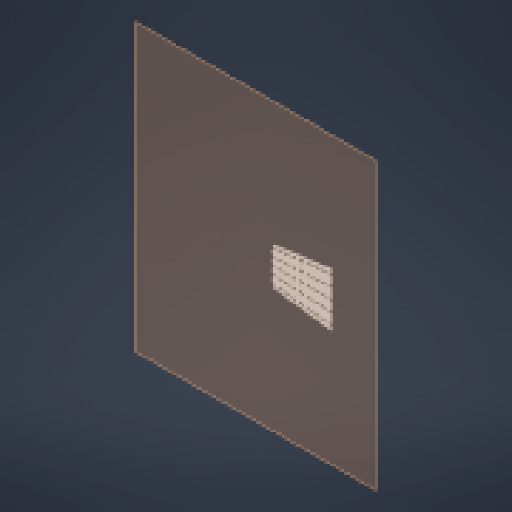
# Autodesk Inventor part: PCB
Saved by Autodesk Inventor 2023 (Build 270158000, 158)
## iProperties
Created: 2022-07-05
Part Number: PCB
Material: Generic
Document SubType Name: Modeling
Designer: FizzyApple12
Density: 1 g/cm^3
Appearance: Default
Author: FizzyApple12
Autodesk Inventor part; units mm, degrees
(part 1 of 2)
ref_plane "YZ Plane" through (0, 0, 0) normal (1, 0, 0) x (0, 1, 0)
ref_plane "XZ Plane" through (0, 0, 0) normal (0, 1, 0) x (-1, 0, 0)
ref_plane "XY Plane" through (0, 0, 0) normal (0, 0, 1) x (1, 0, 0)
ref_plane "Work Plane1" through (0, 0, 0) normal (0, 0, 1) x (1, 0, 0)
sketch "Sketch1" plane through (0, 0, 0) normal (0, 0, 1) x (1, 0, 0)
  line L0 (-101.355, 3.175) -> (-101.355, -3.175) construction
  line L1 (-101.355, -3.175) -> (-123.1468, -3.175) construction
  line L2 (-123.1468, -3.175) -> (-123.1468, 3.175) construction
  line L3 (-123.1468, 3.175) -> (-101.355, 3.175) construction
  line L4 (-101.2199, -3.175) -> (-101.2199, 3.175) construction
  line L5 (-101.2199, 3.175) -> (-5.5562, 3.175) construction
  line L6 (-5.5562, 3.175) -> (-5.5562, -3.175) construction
  line L7 (-5.5562, -3.175) -> (-101.2199, -3.175) construction
  line L8 (120.7237, 3.175) -> (120.7237, -3.175) construction
  line L9 (120.7237, -3.175) -> (5.5563, -3.175) construction
  line L10 (5.5563, -3.175) -> (5.5563, 3.175) construction
  line L11 (5.5563, 3.175) -> (120.7237, 3.175) construction
  line L12 (127.5011, 3.175) -> (127.5011, -3.175) construction
  line L13 (127.5011, -3.175) -> (124.6594, -3.175) construction
  line L14 (124.6594, -3.175) -> (124.6594, 3.175) construction
  line L15 (124.6594, 3.175) -> (127.5011, 3.175) construction
  line L16 (-119.8652, 80.4661) -> (-119.8652, 69.6849) construction
  line L17 (-119.8652, 69.6849) -> (-123.5942, 69.2692) construction
  line L18 (-123.5942, 69.2692) -> (-123.5942, 79.942) construction
  line L19 (-123.5942, 79.942) -> (-119.8652, 80.4661) construction
  line L20 (-119.8652, 63.1931) -> (-119.8652, 36.045) construction
  line L21 (-119.8652, 36.045) -> (-123.5942, 35.8394) construction
  line L22 (-123.5942, 35.8394) -> (-123.5942, 62.7773) construction
  line L23 (-123.5942, 62.7773) -> (-119.8652, 63.1931) construction
  line L24 (-119.8652, 29.66) -> (-119.8652, 3.175) construction
  line L25 (-119.8652, 3.175) -> (-123.5942, 3.175) construction
  line L26 (-123.5942, 3.175) -> (-123.5942, 29.4545) construction
  line L27 (-123.5942, 29.4545) -> (-119.8652, 29.66) construction
  line L28 (-119.8652, -3.175) -> (-119.8652, -29.66) construction
  line L29 (-119.8652, -29.66) -> (-123.5942, -29.4545) construction
  line L30 (-123.5942, -29.4545) -> (-123.5942, -3.175) construction
  line L31 (-123.5942, -3.175) -> (-119.8652, -3.175) construction
  line L32 (-119.8652, -36.045) -> (-119.8652, -63.1931) construction
  line L33 (-119.8652, -63.1931) -> (-123.5942, -62.7773) construction
  line L34 (-123.5942, -62.7773) -> (-123.5942, -35.8394) construction
  line L35 (-123.5942, -35.8394) -> (-119.8652, -36.045) construction
  line L36 (-119.8652, -69.6849) -> (-119.8652, -80.4661) construction
  line L37 (-119.8652, -80.4661) -> (-123.5942, -79.942) construction
  line L38 (-123.5942, -79.942) -> (-123.5942, -69.2692) construction
  line L39 (-123.5942, -69.2692) -> (-119.8652, -69.6849) construction
  line L40 (-109.6354, -30.2239) -> (-110.9009, -36.5392) construction
  line L41 (-110.9009, -36.5392) -> (-123.1468, -35.8641) construction
  line L42 (-123.1468, -35.8641) -> (-123.1468, -29.4791) construction
  line L43 (-123.1468, -29.4791) -> (-109.6354, -30.2239) construction
  line L44 (-104.0884, -30.5297) -> (-105.3539, -36.8449) construction
  line L45 (-105.3539, -36.8449) -> (-109.4238, -36.6206) construction
  line L46 (-109.4238, -36.6206) -> (-109.4238, -30.2356) construction
  line L47 (-109.4238, -30.2356) -> (-104.0884, -30.5297) construction
  line L48 (-101.2199, -37.0728) -> (-101.2199, -30.6879) construction
  line L49 (-101.2199, -30.6879) -> (-6.4561, -35.9117) construction
  line L50 (-6.4561, -35.9117) -> (-6.8056, -42.2774) construction
  line L51 (-6.8056, -42.2774) -> (-101.2199, -37.0728) construction
  line L52 (118.4505, -42.7972) -> (118.5665, -49.1886) construction
  line L53 (118.5665, -49.1886) -> (4.2901, -42.8891) construction
  line L54 (4.2901, -42.8891) -> (4.6396, -36.5234) construction
  line L55 (4.6396, -36.5234) -> (118.4505, -42.7972) construction
  line L56 (-115.3903, -68.5048) -> (-116.0414, -70.1112) construction
  line L57 (-116.0414, -70.1112) -> (-123.1468, -69.3191) construction
  line L58 (-123.1468, -69.3191) -> (-123.1468, -62.8272) construction
  line L59 (-123.1468, -62.8272) -> (-115.3903, -63.6919) construction
  line L60 (-115.3903, -63.6919) -> (-115.3903, -68.5048) construction
  line L61 (-106.228, -71.2052) -> (-103.7108, -64.994) construction
  line L62 (-103.7108, -64.994) -> (-7.378, -75.7333) construction
  line L63 (-7.378, -75.7333) -> (-8.0816, -82.1467) construction
  line L64 (-8.0816, -82.1467) -> (-106.228, -71.2052) construction
  line L65 (121.8551, -96.6323) -> (123.9264, -90.3713) construction
  line L66 (123.9264, -90.3713) -> (132.9258, -91.3746) construction
  line L67 (132.9258, -91.3746) -> (132.9258, -93.8676) construction
  line L68 (132.9258, -93.8676) -> (131.3752, -97.6936) construction
  line L69 (131.3752, -97.6936) -> (121.8551, -96.6323) construction
  line L70 (119.8868, -95.8185) -> (119.9083, -96.4152) construction
  line L71 (119.9083, -96.4152) -> (119.6563, -96.3871) construction
  line L72 (119.6563, -96.3871) -> (119.8868, -95.8185) construction
  line L73 (110.999, -88.9302) -> (110.999, -95.422) construction
  line L74 (110.999, -95.422) -> (-1.3664, -82.8953) construction
  line L75 (-1.3664, -82.8953) -> (-0.6628, -76.4819) construction
  line L76 (-0.6628, -76.4819) -> (110.999, -88.9302) construction
  line L77 (132.9258, -115.9918) -> (132.9258, -119.2788) construction
  line L78 (132.9258, -119.2788) -> (129.106, -118.742) construction
  line L79 (129.106, -118.742) -> (130.6728, -115.6752) construction
  line L80 (130.6728, -115.6752) -> (132.9258, -115.9918) construction
  line L81 (117.7113, -116.5113) -> (117.4113, -117.0985) construction
  line L82 (117.4113, -117.0985) -> (69.7285, -110.3974) construction
  ellipse E0 centre (66.7779, -107.4466) end of major axis (64.6445, -122.6275) minor radius 3.3782 (69.7285, -110.3974) -> (70.2228, -107.1799) ccw construction
  line L83 (70.2228, -107.1799) -> (117.7113, -113.8536) construction
  line L84 (117.7113, -113.8536) -> (117.7113, -116.5113) construction
  line L85 (-122.3603, -80.1155) -> (-123.1468, -81.6549) construction
  line L86 (-123.1468, -81.6549) -> (-123.1468, -80.0049) construction
  line L87 (-123.1468, -80.0049) -> (-122.3603, -80.1155) construction
  line L88 (-107.9322, -85.4301) -> (-107.9322, -82.1431) construction
  line L89 (-107.9322, -82.1431) -> (-61.1887, -88.7121) construction
  ellipse E1 centre (-59.8413, -98.3515) end of major axis (-61.9747, -113.5324) minor radius 3.3782 (-61.1887, -88.7121) -> (-62.0608, -91.8766) ccw construction
  line L90 (-62.0608, -91.8766) -> (-107.9322, -85.4301) construction
  line L91 (63.1283, -109.4699) -> (-55.9232, -92.7391) construction
  ellipse E2 centre (-59.8413, -98.3515) end of major axis (-61.9747, -113.5324) minor radius 3.3782 (-55.9232, -92.7391) -> (-55.8893, -89.4569) ccw construction
  line L92 (-55.8893, -89.4569) -> (63.54, -106.2407) construction
  ellipse E3 centre (66.7779, -107.4466) end of major axis (64.6445, -122.6275) minor radius 3.3782 (63.54, -106.2407) -> (63.1283, -109.4699) ccw construction
  line L93 (-110.9009, 36.5392) -> (-109.6354, 30.2239) construction
  line L94 (-109.6354, 30.2239) -> (-123.1468, 29.4791) construction
  line L95 (-123.1468, 29.4791) -> (-123.1468, 35.8641) construction
  line L96 (-123.1468, 35.8641) -> (-110.9009, 36.5392) construction
  line L97 (-105.3539, 36.8449) -> (-104.0884, 30.5297) construction
  line L98 (-104.0884, 30.5297) -> (-109.4238, 30.2356) construction
  line L99 (-109.4238, 30.2356) -> (-109.4238, 36.6206) construction
  line L100 (-109.4238, 36.6206) -> (-105.3539, 36.8449) construction
  line L101 (-101.2199, 30.6879) -> (-101.2199, 37.0728) construction
  line L102 (-101.2199, 37.0728) -> (-6.8056, 42.2774) construction
  line L103 (-6.8056, 42.2774) -> (-6.4561, 35.9117) construction
  line L104 (-6.4561, 35.9117) -> (-101.2199, 30.6879) construction
  line L105 (118.5665, 49.1886) -> (118.4505, 42.7972) construction
  line L106 (118.4505, 42.7972) -> (4.6396, 36.5234) construction
  line L107 (4.6396, 36.5234) -> (4.2901, 42.8891) construction
  line L108 (4.2901, 42.8891) -> (118.5665, 49.1886) construction
  line L109 (-116.0414, 70.1112) -> (-115.3903, 68.5048) construction
  line L110 (-115.3903, 68.5048) -> (-115.3903, 63.6919) construction
  line L111 (-115.3903, 63.6919) -> (-123.1468, 62.8272) construction
  line L112 (-123.1468, 62.8272) -> (-123.1468, 69.3191) construction
  line L113 (-123.1468, 69.3191) -> (-116.0414, 70.1112) construction
  line L114 (-103.7108, 64.994) -> (-106.228, 71.2052) construction
  line L115 (-106.228, 71.2052) -> (-8.0816, 82.1467) construction
  line L116 (-8.0816, 82.1467) -> (-7.378, 75.7333) construction
  line L117 (-7.378, 75.7333) -> (-103.7108, 64.994) construction
  line L118 (123.9264, 90.3713) -> (121.8551, 96.6323) construction
  line L119 (121.8551, 96.6323) -> (131.3752, 97.6936) construction
  line L120 (131.3752, 97.6936) -> (132.9258, 93.8676) construction
  line L121 (132.9258, 93.8676) -> (132.9258, 91.3746) construction
  line L122 (132.9258, 91.3746) -> (123.9264, 90.3713) construction
  line L123 (119.9083, 96.4152) -> (119.8868, 95.8185) construction
  line L124 (119.8868, 95.8185) -> (119.6563, 96.3871) construction
  line L125 (119.6563, 96.3871) -> (119.9083, 96.4152) construction
  line L126 (110.999, 95.422) -> (110.999, 88.9302) construction
  line L127 (110.999, 88.9302) -> (-0.6628, 76.4819) construction
  line L128 (-0.6628, 76.4819) -> (-1.3664, 82.8953) construction
  line L129 (-1.3664, 82.8953) -> (110.999, 95.422) construction
  line L130 (132.9258, 119.2788) -> (132.9258, 115.9918) construction
  line L131 (132.9258, 115.9918) -> (130.6728, 115.6752) construction
  line L132 (130.6728, 115.6752) -> (129.106, 118.742) construction
  line L133 (129.106, 118.742) -> (132.9258, 119.2788) construction
  line L134 (117.4113, 117.0985) -> (117.7113, 116.5113) construction
  line L135 (117.7113, 116.5113) -> (117.7113, 113.8536) construction
  line L136 (117.7113, 113.8536) -> (70.2228, 107.1799) construction
  ellipse E4 centre (66.7779, 107.4466) end of major axis (64.6445, 122.6275) minor radius 3.3782 (70.2228, 107.1799) -> (69.7285, 110.3974) ccw construction
  line L137 (69.7285, 110.3974) -> (117.4113, 117.0985) construction
  line L138 (-123.1468, 81.6549) -> (-122.3603, 80.1155) construction
  line L139 (-122.3603, 80.1155) -> (-123.1468, 80.0049) construction
  line L140 (-123.1468, 80.0049) -> (-123.1468, 81.6549) construction
  line L141 (-107.9322, 82.1431) -> (-107.9322, 85.4301) construction
  line L142 (-107.9322, 85.4301) -> (-62.0608, 91.8766) construction
  ellipse E5 centre (-59.8413, 98.3515) end of major axis (-61.9747, 113.5324) minor radius 3.3782 (-62.0608, 91.8766) -> (-61.1887, 88.7121) ccw construction
  line L143 (-61.1887, 88.7121) -> (-107.9322, 82.1431) construction
  line L144 (63.54, 106.2407) -> (-55.8893, 89.4569) construction
  ellipse E6 centre (-59.8413, 98.3515) end of major axis (-61.9747, 113.5324) minor radius 3.3782 (-55.8893, 89.4569) -> (-55.9232, 92.7391) ccw construction
  line L145 (-55.9232, 92.7391) -> (63.1283, 109.4699) construction
  ellipse E7 centre (66.7779, 107.4466) end of major axis (64.6445, 122.6275) minor radius 3.3782 (63.1283, 109.4699) -> (63.54, 106.2407) ccw construction
  line L146 (0.1826, -83.068) -> (3.9116, -83.4837) construction
  line L147 (3.9116, -83.4837) -> (3.9116, -97.8609) construction
  line L148 (3.9116, -97.8609) -> (0.1826, -97.3369) construction
  line L149 (0.1826, -97.3369) -> (0.1826, -83.068) construction
  line L150 (3.9116, 83.4837) -> (0.1826, 83.068) construction
  line L151 (0.1826, 83.068) -> (0.1826, 97.3369) construction
  line L152 (0.1826, 97.3369) -> (3.9116, 97.8609) construction
  line L153 (3.9116, 97.8609) -> (3.9116, 83.4837) construction
  line L154 (3.9116, 45.8053) -> (0.1826, 45.5997) construction
  line L155 (0.1826, 45.5997) -> (0.1826, 76.5762) construction
  line L156 (0.1826, 76.5762) -> (3.9116, 76.9919) construction
  line L157 (3.9116, 76.9919) -> (3.9116, 45.8053) construction
  line L158 (3.9116, 6.096) -> (0.1826, 6.096) construction
  line L159 (0.1826, 6.096) -> (0.1826, 33.3406) construction
  line L160 (0.1826, 33.3406) -> (3.9116, 33.5461) construction
  line L161 (3.9116, 33.5461) -> (3.9116, 6.096) construction
  line L162 (3.9116, -33.5461) -> (0.1826, -33.3406) construction
  line L163 (0.1826, -33.3406) -> (0.1826, -6.096) construction
  line L164 (0.1826, -6.096) -> (3.9116, -6.096) construction
  line L165 (3.9116, -6.096) -> (3.9116, -33.5461) construction
  line L166 (0.1826, -45.5997) -> (3.9116, -45.8053) construction
  line L167 (3.9116, -45.8053) -> (3.9116, -76.9919) construction
  line L168 (3.9116, -76.9919) -> (0.1826, -76.5762) construction
  line L169 (0.1826, -76.5762) -> (0.1826, -45.5997) construction
  line L170 (129.6442, 43.4142) -> (133.3733, 43.6198) construction
  line L171 (133.3733, 43.6198) -> (133.3733, 3.175) construction
  line L172 (133.3733, 3.175) -> (133.2928, 3.175) construction
  ellipse E8 centre (131.0926, 0) end of major axis (137.5337, 0) minor radius 3.3782 (133.2928, 3.175) -> (129.6442, 3.2917) ccw construction
  line L173 (129.6442, 3.2917) -> (129.6442, 43.4142) construction
  line L174 (133.3733, -43.6198) -> (129.6442, -43.4142) construction
  line L175 (129.6442, -43.4142) -> (129.6442, -3.2917) construction
  ellipse E9 centre (131.0926, 0) end of major axis (137.5337, 0) minor radius 3.3782 (129.6442, -3.2917) -> (133.2928, -3.175) ccw construction
  line L176 (133.2928, -3.175) -> (133.3733, -3.175) construction
  line L177 (133.3733, -3.175) -> (133.3733, -43.6198) construction
  line L178 (133.3733, -91.4245) -> (129.6442, -91.0088) construction
  line L179 (129.6442, -91.0088) -> (129.6442, -49.7992) construction
  line L180 (129.6442, -49.7992) -> (133.3733, -50.0048) construction
  line L181 (133.3733, -50.0048) -> (133.3733, -91.4245) construction
  line L182 (129.6442, 91.0088) -> (133.3733, 91.4245) construction
  line L183 (133.3733, 91.4245) -> (133.3733, 50.0048) construction
  line L184 (133.3733, 50.0048) -> (129.6442, 49.7992) construction
  line L185 (129.6442, 49.7992) -> (129.6442, 91.0088) construction
  line L186 (133.3733, 116.0547) -> (133.3733, 105.7455) construction
  ellipse E10 centre (131.0926, 102.5862) end of major axis (137.5337, 102.5862) minor radius 3.3782 (133.3733, 105.7455) -> (129.6442, 105.8778) ccw construction
  line L187 (129.6442, 105.8778) -> (129.6442, 115.5306) construction
  line L188 (129.6442, 115.5306) -> (133.3733, 116.0547) construction
  line L189 (133.3733, -92.7634) -> (133.3733, -99.4268) construction
  ellipse E11 centre (131.0926, -102.5862) end of major axis (137.5337, -102.5862) minor radius 3.3782 (133.3733, -99.4268) -> (129.6442, -99.2945) ccw construction
  line L190 (129.6442, -99.2945) -> (129.6442, -97.5006) construction
  line L191 (129.6442, -97.5006) -> (131.3752, -97.6936) construction
  line L192 (131.3752, -97.6936) -> (133.3733, -92.7634) construction
  line L193 (133.3733, -105.7455) -> (133.3733, -116.0547) construction
  line L194 (133.3733, -116.0547) -> (129.6442, -115.5306) construction
  line L195 (129.6442, -115.5306) -> (129.6442, -105.8778) construction
  ellipse E12 centre (131.0926, -102.5862) end of major axis (137.5337, -102.5862) minor radius 3.3782 (129.6442, -105.8778) -> (133.3733, -105.7455) ccw construction
  line L196 (131.3752, 97.6936) -> (129.6442, 97.5006) construction
  line L197 (129.6442, 97.5006) -> (129.6442, 99.2945) construction
  ellipse E13 centre (131.0926, 102.5862) end of major axis (137.5337, 102.5862) minor radius 3.3782 (129.6442, 99.2945) -> (133.3733, 99.4268) ccw construction
  line L198 (133.3733, 99.4268) -> (133.3733, 92.7634) construction
  line L199 (133.3733, 92.7634) -> (131.3752, 97.6936) construction
  line L200 (-119.8652, 29.66) -> (129.6442, 43.4142)
  line L201 (-119.8652, -36.045) -> (129.6442, -49.7992)
  line L202 (-119.8652, -29.66) -> (129.6442, -43.4142)
  line L203 (-119.8652, 3.175) -> (129.6442, 3.175)
  line L204 (-119.8652, -3.175) -> (129.6442, -3.175)
  line L205 (-119.8652, 36.045) -> (129.6442, 49.7992)
  line L206 (-119.8652, -69.6849) -> (129.6442, -97.5006)
  line L207 (-119.8652, -63.1931) -> (129.6442, -91.0088)
  line L208 (-119.8652, 63.1931) -> (129.6442, 91.0088)
  line L209 (-119.8652, 69.6849) -> (129.6442, 97.5006)
  line L210 (129.6442, 43.4142) -> (129.6442, 3.175)
  line L211 (129.6442, 91.0088) -> (129.6442, 49.7992)
  line L212 (129.6442, -3.175) -> (129.6442, -43.4142)
  line L213 (129.6442, -49.7992) -> (129.6442, -91.0088)
  line L214 (-119.8652, -36.045) -> (-119.8652, -63.1931)
  line L215 (-119.8652, 29.66) -> (-119.8652, 3.175)
  line L216 (-119.8652, -3.175) -> (-119.8652, -29.66)
  line L217 (-119.8652, 63.1931) -> (-119.8652, 36.045)
  line L218 (129.6442, -115.5306) -> (-119.8652, -80.4661)
  line L219 (129.6442, 115.5306) -> (-119.8652, 80.4661)
  line L220 (129.6442, 115.5306) -> (129.6442, 97.5006)
  line L221 (-119.8652, -80.4661) -> (-119.8652, -69.6849)
  line L222 (129.6442, -115.5306) -> (129.6442, -97.5006)
  line L223 (0.1826, 97.3369) -> (0.1826, -97.3369)
  line L224 (3.9116, 97.8609) -> (3.9116, -97.8609)
  line L225 (-119.8652, 80.4661) -> (-119.8652, 69.6849)
  point P0 (0, 0)
  point P1 (4.8895, -42.9221)
  point P2 (4.8895, -36.5371)
  point P3 (4.8895, -77.1009)
  point P4 (4.8895, -83.5928)
  point P5 (4.8895, -3.175)
  point P6 (4.8895, 3.175)
  point P7 (4.8895, 42.9221)
  point P8 (4.8895, 77.1009)
  point P9 (4.8895, 83.5928)
  point P10 (129.6442, -70.404)
  point P11 (129.6442, 70.404)
  point P12 (129.6442, 23.2946)
  point P13 (129.6442, -23.2946)
  point P14 (-119.8652, 49.619)
  point P15 (-119.8652, 16.4175)
  point P16 (-119.8652, -16.4175)
  point P17 (-119.8652, -49.619)
  point P18 (4.8895, -97.9984)
  point P19 (4.8895, 97.9984)
  point P20 (129.6442, 106.5156)
  point P21 (129.6442, -106.5156)
  point P22 (-119.8652, -75.0755)
  point P23 (0.1826, 0)
  point P24 (3.9116, 0)
  point P25 (-119.8652, 75.0755)
  point P26 (3.9116, 83.4837)
  point P27 (3.9116, 76.9919)
  point P28 (3.9116, 42.8682)
  point P29 (3.9116, 36.4832)
  point P30 (3.9116, 3.175)
  point P31 (3.9116, -3.175)
  point P32 (3.9116, -36.4832)
  point P33 (3.9116, -42.8682)
  point P34 (3.9116, -76.9919)
  point P35 (3.9116, -83.4837)
  point P36 (0.1826, -83.068)
  point P37 (0.1826, -76.5762)
  point P38 (0.1826, -42.6626)
  point P39 (0.1826, -36.2777)
  point P40 (0.1826, -3.175)
  point P41 (0.1826, 3.175)
  point P42 (0.1826, 36.2777)
  point P43 (0.1826, 42.6626)
  point P44 (0.1826, 76.5762)
  point P45 (0.1826, 83.068)
  constraints: 452 end point, 70 point on line, 70 vertical, 33 midpoint, 26 collinear, 14 horizontal, 398 other
extrude "Extrusion1" add sketch "Sketch1" against normal blind 1.6 contours L200 L223 L203 L215 | L200 L210 L203 L224 | L205 L217 L208 L223 | L224 L208 L211 L205 | L223 L202 L216 L204 | L204 L212 L202 L224 | L209 L225 L219 L223 | L224 L219 L220 L209 | L223 L207 L214 L201 | L201 L213 L207 L224 | L223 L218 L221 L206 | L206 L222 L218 L224
sketch "Sketch2" plane through (0, 0, -1.6) normal (0, 0, -1) x (-1, 0, 0)
  line L0 (-4.8972, -83.8832) -> (-1.1682, -83.4675) construction
  line L1 (-1.1682, -83.4675) -> (-1.1682, -97.8404) construction
  line L2 (-1.1682, -97.8404) -> (-4.8972, -98.3645) construction
  line L3 (-4.8972, -98.3645) -> (-4.8972, -83.8832) construction
  line L4 (-1.1682, 83.4675) -> (-4.8972, 83.8832) construction
  line L5 (-4.8972, 83.8832) -> (-4.8972, 98.3645) construction
  line L6 (-4.8972, 98.3645) -> (-1.1682, 97.8404) construction
  line L7 (-1.1682, 97.8404) -> (-1.1682, 83.4675) construction
  line L8 (-1.1682, 45.7972) -> (-2.4514, 45.868) construction
  line L9 (-2.4514, 45.868) -> (-3.0335, 42.963) construction
  line L10 (-3.0335, 42.963) -> (-4.8972, 43.0657) construction
  line L11 (-4.8972, 43.0657) -> (-4.8972, 77.3913) construction
  line L12 (-4.8972, 77.3913) -> (-1.1682, 76.9756) construction
  line L13 (-1.1682, 76.9756) -> (-1.1682, 45.7972) construction
  line L14 (-1.1682, 6.096) -> (-4.8972, 6.096) construction
  line L15 (-4.8972, 6.096) -> (-4.8972, 36.6807) construction
  line L16 (-4.8972, 36.6807) -> (-4.2991, 36.6478) construction
  line L17 (-4.2991, 36.6478) -> (-4.8812, 33.7428) construction
  line L18 (-4.8812, 33.7428) -> (-1.1682, 33.5381) construction
  line L19 (-1.1682, 33.5381) -> (-1.1682, 6.096) construction
  line L20 (-1.1682, -33.5381) -> (-4.8812, -33.7428) construction
  line L21 (-4.8812, -33.7428) -> (-4.2991, -36.6478) construction
  line L22 (-4.2991, -36.6478) -> (-4.8972, -36.6807) construction
  line L23 (-4.8972, -36.6807) -> (-4.8972, -6.096) construction
  line L24 (-4.8972, -6.096) -> (-1.1682, -6.096) construction
  line L25 (-1.1682, -6.096) -> (-1.1682, -33.5381) construction
  line L26 (-4.8972, -43.0657) -> (-3.0335, -42.963) construction
  line L27 (-3.0335, -42.963) -> (-2.4514, -45.868) construction
  line L28 (-2.4514, -45.868) -> (-1.1682, -45.7972) construction
  line L29 (-1.1682, -45.7972) -> (-1.1682, -76.9756) construction
  line L30 (-1.1682, -76.9756) -> (-4.8972, -77.3913) construction
  line L31 (-4.8972, -77.3913) -> (-4.8972, -43.0657) construction
  line L32 (118.8796, -80.9696) -> (118.8796, -70.0844) construction
  line L33 (118.8796, -70.0844) -> (122.6086, -69.6686) construction
  line L34 (122.6086, -69.6686) -> (122.6086, -80.4456) construction
  line L35 (122.6086, -80.4456) -> (118.8796, -80.9696) construction
  line L36 (118.8796, -63.5925) -> (118.8796, -36.2425) construction
  line L37 (118.8796, -36.2425) -> (122.6086, -36.037) construction
  line L38 (122.6086, -36.037) -> (122.6086, -63.1768) construction
  line L39 (122.6086, -63.1768) -> (118.8796, -63.5925) construction
  line L40 (118.8796, -29.8575) -> (118.8796, -3.175) construction
  line L41 (118.8796, -3.175) -> (122.6086, -3.175) construction
  line L42 (122.6086, -3.175) -> (122.6086, -29.652) construction
  line L43 (122.6086, -29.652) -> (118.8796, -29.8575) construction
  line L44 (118.8796, 3.175) -> (118.8796, 29.8575) construction
  line L45 (118.8796, 29.8575) -> (122.6086, 29.652) construction
  line L46 (122.6086, 29.652) -> (122.6086, 3.175) construction
  line L47 (122.6086, 3.175) -> (118.8796, 3.175) construction
  line L48 (118.8796, 36.2425) -> (118.8796, 63.5925) construction
  line L49 (118.8796, 63.5925) -> (122.6086, 63.1768) construction
  line L50 (122.6086, 63.1768) -> (122.6086, 36.037) construction
  line L51 (122.6086, 36.037) -> (118.8796, 36.2425) construction
  line L52 (118.8796, 70.0844) -> (118.8796, 80.9696) construction
  line L53 (118.8796, 80.9696) -> (122.6086, 80.4456) construction
  line L54 (122.6086, 80.4456) -> (122.6086, 69.6686) construction
  line L55 (122.6086, 69.6686) -> (118.8796, 70.0844) construction
  line L56 (-133.9114, 116.4953) -> (-133.9114, 116.5191) construction
  line L57 (-133.9114, 116.5191) -> (-132.356, 119.5637) construction
  line L58 (-132.356, 119.5637) -> (-126.5086, 118.742) construction
  line L59 (-126.5086, 118.742) -> (-128.0754, 115.6752) construction
  line L60 (-128.0754, 115.6752) -> (-133.9114, 116.4953) construction
  line L61 (-116.3807, 114.0317) -> (-114.8139, 117.0985) construction
  line L62 (-114.8139, 117.0985) -> (-68.9221, 110.6491) construction
  ellipse E0 centre (-67.7635, 100.4333) end of major axis (-65.6301, 115.6142) minor radius 3.3782 (-68.9221, 110.6491) -> (-69.84, 107.4911) ccw construction
  line L63 (-69.84, 107.4911) -> (-116.3807, 114.0317) construction
  line L64 (112.9131, 81.8081) -> (112.9131, 85.0951) construction
  line L65 (112.9131, 85.0951) -> (114.8297, 84.8258) construction
  line L66 (114.8297, 84.8258) -> (113.263, 81.759) construction
  line L67 (113.263, 81.759) -> (112.9131, 81.8081) construction
  line L68 (110.4442, 85.4421) -> (108.8774, 82.3753) construction
  line L69 (108.8774, 82.3753) -> (61.9084, 88.976) construction
  ellipse E1 centre (58.8557, 91.3382) end of major axis (60.9891, 106.5191) minor radius 3.3782 (61.9084, 88.976) -> (62.3748, 92.1975) ccw construction
  line L70 (62.3748, 92.1975) -> (110.4442, 85.4421) construction
  line L71 (55.2701, 89.9089) -> (-63.8222, 106.6454) construction
  ellipse E2 centre (-67.7635, 100.4333) end of major axis (-65.6301, 115.6142) minor radius 3.3782 (-63.8222, 106.6454) -> (-63.8341, 109.9341) ccw construction
  line L72 (-63.8341, 109.9341) -> (55.7098, 93.1341) construction
  ellipse E3 centre (58.8557, 91.3382) end of major axis (60.9891, 106.5191) minor radius 3.3782 (55.7098, 93.1341) -> (55.2701, 89.9089) ccw construction
  line L73 (-134.3589, 43.8173) -> (-130.6298, 43.6118) construction
  line L74 (-130.6298, 43.6118) -> (-130.6298, 3.1873) construction
  ellipse E4 centre (-128.4952, 0) end of major axis (-134.9363, 0) minor radius 3.3782 (-130.6298, 3.1873) -> (-130.6954, 3.175) ccw construction
  line L75 (-130.6954, 3.175) -> (-134.3589, 3.175) construction
  line L76 (-134.3589, 3.175) -> (-134.3589, 43.8173) construction
  line L77 (-130.6298, -43.6118) -> (-134.3589, -43.8173) construction
  line L78 (-134.3589, -43.8173) -> (-134.3589, -3.175) construction
  line L79 (-134.3589, -3.175) -> (-130.6954, -3.175) construction
  ellipse E5 centre (-128.4952, 0) end of major axis (-134.9363, 0) minor radius 3.3782 (-130.6954, -3.175) -> (-130.6298, -3.1873) ccw construction
  line L80 (-130.6298, -3.1873) -> (-130.6298, -43.6118) construction
  line L81 (-130.6298, -91.4082) -> (-131.2951, -91.4824) construction
  line L82 (-131.2951, -91.4824) -> (-130.6298, -93.1238) construction
  line L83 (-130.6298, -93.1238) -> (-130.6298, -99.3989) construction
  ellipse E6 centre (-128.4952, -102.5862) end of major axis (-134.9363, -102.5862) minor radius 3.3782 (-130.6298, -99.3989) -> (-134.3589, -101.1882) ccw construction
  line L84 (-134.3589, -101.1882) -> (-134.3589, -50.2023) construction
  line L85 (-134.3589, -50.2023) -> (-130.6298, -49.9967) construction
  line L86 (-130.6298, -49.9967) -> (-130.6298, -91.4082) construction
  line L87 (-131.2951, 91.4824) -> (-130.6298, 91.4082) construction
  line L88 (-130.6298, 91.4082) -> (-130.6298, 49.9967) construction
  line L89 (-130.6298, 49.9967) -> (-134.3589, 50.2023) construction
  line L90 (-134.3589, 50.2023) -> (-134.3589, 101.1882) construction
  ellipse E7 centre (-128.4952, 102.5862) end of major axis (-134.9363, 102.5862) minor radius 3.3782 (-134.3589, 101.1882) -> (-130.6298, 99.3989) ccw construction
  line L91 (-130.6298, 99.3989) -> (-130.6298, 93.1238) construction
  line L92 (-130.6298, 93.1238) -> (-131.2951, 91.4824) construction
  line L93 (-134.3589, 103.9841) -> (-134.3589, 119.8452) construction
  line L94 (-134.3589, 119.8452) -> (-132.356, 119.5637) construction
  line L95 (-132.356, 119.5637) -> (-133.9227, 116.4969) construction
  line L96 (-133.9227, 116.4969) -> (-130.6298, 116.0342) construction
  line L97 (-130.6298, 116.0342) -> (-130.6298, 105.7735) construction
  ellipse E8 centre (-128.4952, 102.5862) end of major axis (-134.9363, 102.5862) minor radius 3.3782 (-130.6298, 105.7735) -> (-134.3589, 103.9841) ccw construction
  line L98 (-133.9227, -116.4969) -> (-132.356, -119.5637) construction
  line L99 (-132.356, -119.5637) -> (-134.3589, -119.8452) construction
  line L100 (-134.3589, -119.8452) -> (-134.3589, -103.9841) construction
  ellipse E9 centre (-128.4952, -102.5862) end of major axis (-134.9363, -102.5862) minor radius 3.3782 (-134.3589, -103.9841) -> (-130.6298, -105.7735) ccw construction
  line L101 (-130.6298, -105.7735) -> (-130.6298, -116.0342) construction
  line L102 (-130.6298, -116.0342) -> (-133.9227, -116.4969) construction
  line L103 (-133.9114, -116.5191) -> (-133.9114, -116.4953) construction
  line L104 (-133.9114, -116.4953) -> (-128.0754, -115.6752) construction
  line L105 (-128.0754, -115.6752) -> (-126.5086, -118.742) construction
  line L106 (-126.5086, -118.742) -> (-132.356, -119.5637) construction
  line L107 (-132.356, -119.5637) -> (-133.9114, -116.5191) construction
  line L108 (-114.8139, -117.0985) -> (-116.3807, -114.0317) construction
  line L109 (-116.3807, -114.0317) -> (-69.84, -107.4911) construction
  ellipse E10 centre (-67.7635, -100.4333) end of major axis (-65.6301, -115.6142) minor radius 3.3782 (-69.84, -107.4911) -> (-68.9221, -110.6491) ccw construction
  line L110 (-68.9221, -110.6491) -> (-114.8139, -117.0985) construction
  line L111 (112.9131, -85.0951) -> (112.9131, -81.8081) construction
  line L112 (112.9131, -81.8081) -> (113.263, -81.759) construction
  line L113 (113.263, -81.759) -> (114.8297, -84.8258) construction
  line L114 (114.8297, -84.8258) -> (112.9131, -85.0951) construction
  line L115 (108.8774, -82.3753) -> (110.4442, -85.4421) construction
  line L116 (110.4442, -85.4421) -> (62.3748, -92.1975) construction
  ellipse E11 centre (58.8557, -91.3382) end of major axis (60.9891, -106.5191) minor radius 3.3782 (62.3748, -92.1975) -> (61.9084, -88.976) ccw construction
  line L117 (61.9084, -88.976) -> (108.8774, -82.3753) construction
  line L118 (55.7098, -93.1341) -> (-63.8341, -109.9341) construction
  ellipse E12 centre (-67.7635, -100.4333) end of major axis (-65.6301, -115.6142) minor radius 3.3782 (-63.8341, -109.9341) -> (-63.8222, -106.6454) ccw construction
  line L119 (-63.8222, -106.6454) -> (55.2701, -89.9089) construction
  ellipse E13 centre (58.8557, -91.3382) end of major axis (60.9891, -106.5191) minor radius 3.3782 (55.2701, -89.9089) -> (55.7098, -93.1341) ccw construction
  line L120 (118.6387, -70.1112) -> (116.1215, -63.9) construction
  line L121 (116.1215, -63.9) -> (122.1611, -63.2267) construction
  line L122 (122.1611, -63.2267) -> (122.1611, -69.7185) construction
  line L123 (122.1611, -69.7185) -> (118.6387, -70.1112) construction
  line L124 (106.3082, -64.994) -> (108.4382, -70.2499) construction
  line L125 (108.4382, -70.2499) -> (108.4382, -71.2484) construction
  line L126 (108.4382, -71.2484) -> (8.0974, -82.4345) construction
  line L127 (8.0974, -82.4345) -> (7.3938, -76.0211) construction
  line L128 (7.3938, -76.0211) -> (106.3082, -64.994) construction
  line L129 (-119.5762, -90.1759) -> (-117.059, -96.3871) construction
  line L130 (-117.059, -96.3871) -> (-130.6298, -97.9001) construction
  line L131 (-130.6298, -97.9001) -> (-130.6298, -93.1238) construction
  line L132 (-130.6298, -93.1238) -> (-131.2951, -91.4824) construction
  line L133 (-131.2951, -91.4824) -> (-121.9637, -90.4421) construction
  line L134 (-121.9637, -90.4421) -> (-121.0923, -93.0761) construction
  line L135 (-121.0923, -93.0761) -> (-120.9934, -90.3339) construction
  line L136 (-120.9934, -90.3339) -> (-119.5762, -90.1759) construction
  line L137 (-111.9846, -95.8215) -> (-111.9846, -89.3296) construction
  line L138 (-111.9846, -89.3296) -> (0.6787, -76.7697) construction
  line L139 (0.6787, -76.7697) -> (1.3823, -83.1831) construction
  line L140 (1.3823, -83.1831) -> (-111.9846, -95.8215) construction
  line L141 (113.4983, -36.5392) -> (112.2328, -30.2239) construction
  line L142 (112.2328, -30.2239) -> (122.1611, -29.6766) construction
  line L143 (122.1611, -29.6766) -> (122.1611, -36.0616) construction
  line L144 (122.1611, -36.0616) -> (113.4983, -36.5392) construction
  line L145 (107.9513, -36.8449) -> (106.6858, -30.5297) construction
  line L146 (106.6858, -30.5297) -> (108.4382, -30.4331) construction
  line L147 (108.4382, -30.4331) -> (108.4382, -36.8181) construction
  line L148 (108.4382, -36.8181) -> (107.9513, -36.8449) construction
  line L149 (100.2343, -30.8854) -> (100.2343, -37.2703) construction
  line L150 (100.2343, -37.2703) -> (4.6348, -42.5403) construction
  line L151 (4.6348, -42.5403) -> (4.2853, -36.1746) construction
  line L152 (4.2853, -36.1746) -> (100.2343, -30.8854) construction
  line L153 (-132.9575, -43.7401) -> (-131.692, -50.0553) construction
  line L154 (-131.692, -50.0553) -> (-133.9114, -50.1776) construction
  line L155 (-133.9114, -50.1776) -> (-133.9114, -43.7927) construction
  line L156 (-133.9114, -43.7927) -> (-132.9575, -43.7401) construction
  line L157 (-119.6511, -49.3915) -> (-119.8613, -48.3425) construction
  line L158 (-119.8613, -48.3425) -> (-119.7645, -43.0128) construction
  line L159 (-119.7645, -43.0128) -> (-2.4609, -36.5464) construction
  line L160 (-2.4609, -36.5464) -> (-2.1114, -42.9122) construction
  line L161 (-2.1114, -42.9122) -> (-119.6511, -49.3915) construction
  line L162 (109.5299, -3.175) -> (109.5299, 3.175) construction
  line L163 (109.5299, 3.175) -> (122.1611, 3.175) construction
  line L164 (122.1611, 3.175) -> (122.1611, -3.175) construction
  line L165 (122.1611, -3.175) -> (109.5299, -3.175) construction
  line L166 (103.9524, -3.175) -> (103.9524, 3.175) construction
  line L167 (103.9524, 3.175) -> (108.4382, 3.175) construction
  line L168 (108.4382, 3.175) -> (108.4382, -3.175) construction
  line L169 (108.4382, -3.175) -> (103.9524, -3.175) construction
  line L170 (100.2343, 3.175) -> (100.2343, -3.175) construction
  line L171 (100.2343, -3.175) -> (5.5562, -3.175) construction
  line L172 (5.5562, -3.175) -> (5.5562, 3.175) construction
  line L173 (5.5562, 3.175) -> (100.2343, 3.175) construction
  line L174 (-119.4018, -3.175) -> (-119.4018, 3.175) construction
  line L175 (-119.4018, 3.175) -> (-5.5563, 3.175) construction
  line L176 (-5.5563, 3.175) -> (-5.5563, -3.175) construction
  line L177 (-5.5563, -3.175) -> (-119.4018, -3.175) construction
  line L178 (112.2328, 30.2239) -> (113.4983, 36.5392) construction
  line L179 (113.4983, 36.5392) -> (122.1611, 36.0616) construction
  line L180 (122.1611, 36.0616) -> (122.1611, 29.6766) construction
  line L181 (122.1611, 29.6766) -> (112.2328, 30.2239) construction
  line L182 (106.6858, 30.5297) -> (107.9513, 36.8449) construction
  line L183 (107.9513, 36.8449) -> (108.4382, 36.8181) construction
  line L184 (108.4382, 36.8181) -> (108.4382, 30.4331) construction
  line L185 (108.4382, 30.4331) -> (106.6858, 30.5297) construction
  line L186 (100.2343, 37.2703) -> (100.2343, 30.8854) construction
  line L187 (100.2343, 30.8854) -> (4.2853, 36.1746) construction
  line L188 (4.2853, 36.1746) -> (4.6348, 42.5403) construction
  line L189 (4.6348, 42.5403) -> (100.2343, 37.2703) construction
  line L190 (-131.692, 50.0553) -> (-132.9575, 43.7401) construction
  line L191 (-132.9575, 43.7401) -> (-133.9114, 43.7927) construction
  line L192 (-133.9114, 43.7927) -> (-133.9114, 50.1776) construction
  line L193 (-133.9114, 50.1776) -> (-131.692, 50.0553) construction
  line L194 (-119.8613, 48.3425) -> (-119.6511, 49.3915) construction
  line L195 (-119.6511, 49.3915) -> (-2.1114, 42.9122) construction
  line L196 (-2.1114, 42.9122) -> (-2.4609, 36.5464) construction
  line L197 (-2.4609, 36.5464) -> (-119.7645, 43.0128) construction
  line L198 (-119.7645, 43.0128) -> (-119.8613, 48.3425) construction
  line L199 (116.1215, 63.9) -> (118.6387, 70.1112) construction
  line L200 (118.6387, 70.1112) -> (122.1611, 69.7185) construction
  line L201 (122.1611, 69.7185) -> (122.1611, 63.2267) construction
  line L202 (122.1611, 63.2267) -> (116.1215, 63.9) construction
  line L203 (108.4382, 70.2499) -> (106.3082, 64.994) construction
  line L204 (106.3082, 64.994) -> (7.3938, 76.0211) construction
  line L205 (7.3938, 76.0211) -> (8.0974, 82.4345) construction
  line L206 (8.0974, 82.4345) -> (108.4382, 71.2484) construction
  line L207 (108.4382, 71.2484) -> (108.4382, 70.2499) construction
  line L208 (-117.059, 96.3871) -> (-119.5762, 90.1759) construction
  line L209 (-119.5762, 90.1759) -> (-120.9934, 90.3339) construction
  line L210 (-120.9934, 90.3339) -> (-121.0923, 93.0761) construction
  line L211 (-121.0923, 93.0761) -> (-121.9637, 90.4421) construction
  line L212 (-121.9637, 90.4421) -> (-131.2951, 91.4824) construction
  line L213 (-131.2951, 91.4824) -> (-130.6298, 93.1238) construction
  line L214 (-130.6298, 93.1238) -> (-130.6298, 97.9001) construction
  line L215 (-130.6298, 97.9001) -> (-117.059, 96.3871) construction
  line L216 (-111.9846, 89.3296) -> (-111.9846, 95.8215) construction
  line L217 (-111.9846, 95.8215) -> (1.3823, 83.1831) construction
  line L218 (1.3823, 83.1831) -> (0.6787, 76.7697) construction
  line L219 (0.6787, 76.7697) -> (-111.9846, 89.3296) construction
  line L220 (118.8796, -70.0844) -> (-130.6298, -97.9001)
  line L221 (118.8796, 70.0844) -> (-130.6299, 97.9001)
  line L222 (118.8796, 36.2425) -> (-130.6298, 49.9967)
  line L223 (118.8796, -36.2425) -> (-130.6298, -49.9967)
  line L224 (-4.8972, 98.3645) -> (-4.8972, -98.3645)
  line L225 (118.8796, 80.9696) -> (118.8796, -80.9696)
  line L226 (-1.1682, 97.8404) -> (-1.1682, -97.8404)
  line L227 (-0.1826, 76.5762) -> (-0.1826, 42.6626) construction
  line L228 (-1.1682, 97.8404) -> (-4.8972, 98.3645)
  line L229 (-4.8972, -98.3645) -> (-1.1682, -97.8404)
  line L230 (122.6086, -80.4456) -> (122.6086, 80.4456)
  line L231 (118.8796, 80.9696) -> (122.6086, 80.4456)
  line L232 (118.8796, -80.9696) -> (122.6086, -80.4456)
  line L233 (118.8796, 29.8575) -> (-130.6298, 43.6118)
  line L234 (118.8796, 63.5925) -> (-130.6299, 91.4082)
  line L235 (118.8796, -29.8575) -> (-130.6298, -43.6118)
  line L236 (118.8796, -63.5925) -> (-130.6298, -91.4082)
  line L237 (-130.6299, 97.9001) -> (-130.6299, 91.4082)
  line L238 (-130.6298, 49.9967) -> (-130.6298, 43.6118)
  line L239 (-130.6298, -43.6118) -> (-130.6298, -49.9967)
  line L240 (-130.6298, -91.4082) -> (-130.6298, -97.9001)
  point P0 (0, 0)
  point P1 (-5.8751, -83.9922)
  point P2 (-5.8751, -43.1196)
  point P3 (-5.8751, 43.1196)
  point P4 (-5.8751, 83.9922)
  point P5 (-4.8972, 0)
  point P6 (118.8796, 0)
  point P7 (-1.1682, 0)
  point P8 (-3.0327, -98.1024)
  point P9 (-3.0327, 98.1024)
  point P10 (-1.1682, -42.8602)
  point P11 (-1.1682, -76.9756)
  point P12 (-1.1682, -83.4675)
  point P13 (-1.1682, 83.4675)
  point P14 (-4.8972, 83.8832)
  point P15 (-4.8972, 77.3913)
  point P16 (-4.8972, 43.0657)
  point P17 (-4.8972, 36.6807)
  point P18 (-4.8972, -36.6807)
  point P19 (-4.8972, -43.0657)
  point P20 (-4.8972, -77.3913)
  point P21 (-4.8972, -83.8832)
  point P22 (-1.1682, 42.8602)
  point P23 (-1.1682, 76.9756)
  point P24 (-1.1682, -36.4752)
  point P25 (-1.1682, 36.4752)
  constraints: 480 end point, 66 vertical, 29 point on line, 14 horizontal, 10 midpoint, 9 collinear, 1 parallel, 440 other
extrude "Extrusion2" cut sketch "Sketch2" against normal through all contours L220 L226 L236 L225 | L225 L231 L230 L232 | L226 L229 L224 L220 | L220 L224 L236 L226 | L220 L240 L236 L224 | L236 L224 L223 L226 | L223 L226 L235 L225 | L223 L224 L235 L226 | L223 L239 L235 L224 | L235 L224 L233 L226 | L233 L226 L222 L225 | L233 L224 L222 L226 | L225 L234 L226 L221 | L233 L238 L222 L224 | L222 L224 L234 L226 | L226 L234 L224 L221 | L221 L224 L228 L226 | L224 L234 L237 L221